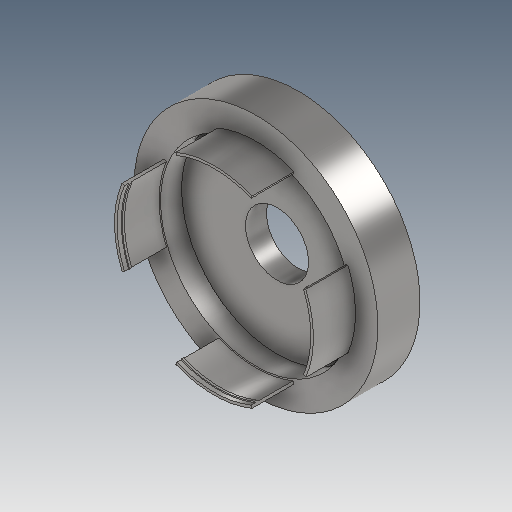
# Autodesk Inventor part: Housing of planetary gearbox
Saved by Autodesk Inventor 2020.3 (Build 243373010, 373A)
## iProperties
Created: 2021-05-05
Part Number: Housing of planetary gearbox
Material: Steel, Alloy
Document SubType Name: Modeling
Designer: marti
Density: 7.73 g/cm^3
Appearance: Semi-Polished
Author: marti
Autodesk Inventor part; units mm, degrees
ref_plane "YZ Plane" through (0, 0, 0) normal (1, 0, 0) x (0, 1, 0)
ref_plane "XZ Plane" through (0, 0, 0) normal (0, 1, 0) x (-1, 0, 0)
sketch "Sketch1" plane through (0, 0, 0) normal (0, 0, 1) x (1, 0, 0)
  circle A0 centre (0, 0) radius 24
  circle A1 centre (0, 0) radius 22.7
  dimension "d0" = 48
  dimension "d1" = 45.4
  constraints: 2 centre point, 2 coincident
  measures "d0" diameter of A0
  measures "d1" diameter of A1
extrude "Extrusion1" add sketch "Sketch1" along normal blind 5
sketch "Sketch2" plane through (0, 0, 0) normal (0, 0, -1) x (-1, 0, 0)
  circle A0 centre (0, 0) radius 24 projected
  circle A1 centre (0, 0) radius 7.5
  dimension "d4" = 15
  constraints: 1 centre point, 1 coincident
  measures "d4" diameter of A1
extrude "Extrusion2" add sketch "Sketch2" along normal blind 5
sketch "Sketch3" plane through (0, 0, 5) normal (0, 0, 1) x (1, 0, 0)
  circle A0 centre (0, 0) radius 22.7 projected
  circle A1 centre (0, 0) radius 24 projected
  arc A2 (8.8209, 21.2954) -> (-8.8209, 21.2954) centre (0, 0) ccw
  arc A3 (9.0505, 21.8498) -> (-9.0505, 21.8498) centre (0, 0) ccw
  circle A4 centre (0, 0) radius 7.5 projected
  line L0 (0, 0) -> (0, 19.001)
  line L1 (-8.8209, 21.2954) -> (-9.0505, 21.8498)
  line L2 (8.8209, 21.2954) -> (9.0505, 21.8498)
  arc A5 (-21.2954, 8.8209) -> (-21.2954, -8.8209) centre (0, 0) ccw
  arc A6 (-21.8498, 9.0505) -> (-21.8498, -9.0505) centre (0, 0) ccw
  line L3 (-21.2954, -8.8209) -> (-21.8498, -9.0505)
  line L4 (-21.2954, 8.8209) -> (-21.8498, 9.0505)
  arc A7 (-8.8209, -21.2954) -> (8.8209, -21.2954) centre (0, 0) ccw
  arc A8 (-9.0505, -21.8498) -> (9.0505, -21.8498) centre (0, 0) ccw
  line L5 (8.8209, -21.2954) -> (9.0505, -21.8498)
  line L6 (-8.8209, -21.2954) -> (-9.0505, -21.8498)
  arc A9 (21.2954, -8.8209) -> (21.2954, 8.8209) centre (0, 0) ccw
  arc A10 (21.8498, -9.0505) -> (21.8498, 9.0505) centre (0, 0) ccw
  line L7 (21.2954, 8.8209) -> (21.8498, 9.0505)
  line L8 (21.2954, -8.8209) -> (21.8498, -9.0505)
  point P0 (-19.001, 0)
  point P1 (0, -19.001)
  point P2 (19.001, 0)
  dimension "d7" = 0.35
  dimension "d8" = 0.35
  dimension "d13" = 360
  constraints: 18 end point, 16 point on circle, 8 centre point, 2 coincident, 1 vertical, 47 other
  measures "d7" radial gap between concentric circles of A0 A2
  measures "d8" radial gap between concentric circles of A1 A3
extrude "Extrusion3" add sketch "Sketch3" along normal blind 10 contours A2 L1 A3 L2 | A5 L3 A6 L4 | A7 L5 A8 L6 | A9 L7 A10 L8
ref_plane "Work Plane2" through (0, 0, 13.75) normal (0, 0, 1) x (1, 0, 0)
sketch "Sketch6" plane through (0, 0, 13.75) normal (0, 0, 1) x (1, 0, 0)
  arc A0 (-8.8209, -21.2954) -> (8.8209, -21.2954) centre (0, 0) ccw projected
  arc A1 (-8.7252, -21.0645) -> (8.7252, -21.0645) centre (0, 0) ccw
  line L0 (-8.7252, -21.0645) -> (-8.8209, -21.2954)
  line L1 (8.7252, -21.0645) -> (8.8209, -21.2954)
  dimension "d19" = 0.25
  constraints: 4 end point, 2 point on circle, 1 centre point
  measures "d19" radial gap between concentric circles of A0 A1
extrude "Extrusion4" add sketch "Sketch6" along normal mid plane 0.5
pattern_circular "Circular Pattern1" count 4 over 360 about axis through (0, 0, -10) along (0, 0, 1) of "Extrusion4"
sketch "Sketch7" plane through (0, 0, -5) normal (0, 0, -1) x (-1, 0, 0)
  circle A0 centre (0, 0) radius 7.5 projected
  circle A1 centre (0, 0) radius 29
  circle A2 centre (0, 0) radius 24 projected
  dimension "d26" = 58
  constraints: 1 centre point, 1 coincident
  measures "d26" diameter of A1
extrude "Extrusion5" add sketch "Sketch7" against normal blind 10 contours A1
sketch "Sketch8" plane through (0, 0, -5) normal (0, 0, -1) x (-1, 0, 0)
  circle A0 centre (17.9207, 17.9207) radius 1.425
  circle A1 centre (17.9207, -17.9207) radius 1.425
  circle A2 centre (-17.9207, -17.9207) radius 1.425
  circle A3 centre (-17.9207, 17.9207) radius 1.425
  point P0 (0, 0)
  point P1 (0, 0)
  constraints: 4 centre point
hole "Hole1" at (17.9207, 17.9207, -5) at (17.9207, -17.9207, -5) at (-17.9207, -17.9207, -5) at (-17.9207, 17.9207, -5) direction (0, 0, 1) diameter 2.459 depth 8.8 counterbore diameter 6 counterbore depth 2 thread size "M3x0.5" class "6H" standard "ISO Metric profile"
equation "\"d10\" = 0.5 * d9"
equation "\"d9\" = 45deg"
body "Solid1"
